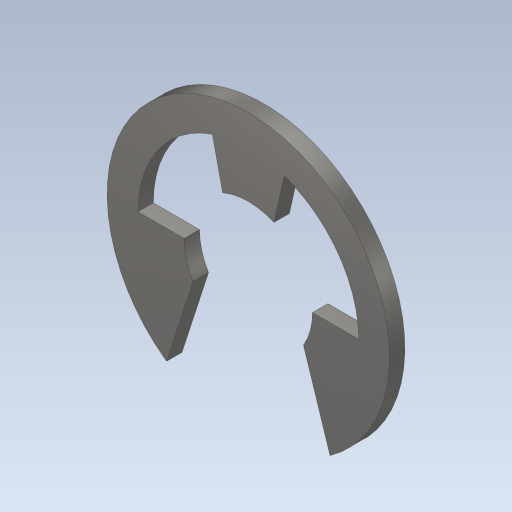
# Autodesk Inventor part: RRING_E_EXT-S-5
Saved by Autodesk Inventor 2024 (Build 280153000, 153)
## iProperties
Created: 2023-10-14
Part Number: RRING_E_EXT-S-5
Material: ステンレス鋼
Catalog Web Link: www.cadenas.de
Description: RRING_E_EXT-Retaining Rings - E
Vendor: MISUMI
Document SubType Name: Modeling
Designer: psAdmin
Manufacturer: MISUMI
Mass: 0.205469 g
Surface Area: 1.19896 cm^2
Volume: 0.0256836 cm^3
Density: 8 g/cm^3
Appearance: 半つや出し
Category: PARTsolutions
Company: MISUMI
PSOL_IDENT_0: {$CADENAS_DATA/23d-libs/misumi/metric/accessories/rring_e_ext.prj},178 {VTYP=3D},{NB=RRING_E_EXT-S-5
PSOL_IDENT_1: },{LINA=RRING_E_EXT-S-5},{NN=RRING_E_EXT},{DATE=08.06.2021 06:39:29},{GEOMDATE=29.08.2013 00:00:00},
PSOL_IDENT_2: {VERSION=},{LINEID=70},{WBVAR=MAT},{WBNUMERIC=}  {NB=RRING_E_EXT-S-5},{LINA=RRING_E_EXT-S-5},{KT=DUM
PSOL_IDENT_3: MY},{PN=RRING_E_EXT-S-5},{TS=RRING_E_EXT},{MAT=-S},{HARD=37~44HRC},{ST=-},{NO=5},{DD=5.0},{DDTOL=0/-
PSOL_IDENT_4: 0.12},{D=11},{DTOL=+0.2/-0.2},{H=4.3},{HTOL=0/-0.30},{TT=0.6},{TTTOL=+0.4/-0.4},{DD1=6~},{LESS=~8},{
PSOL_IDENT_5: DD2=5.0},{DD2TOL=+0.075/0},{MM=0.7},{MMTOL=+0.1/0},{NN=1.2},{MATRR=Steel for Springs},{D1=8.600},{H1=
PSOL_IDENT_6: 2.800},{DEG1=25.400},{DEG2=35.700}
NB: RRING_E_EXT-S-5
NN: 1.2
NT: Retaining Rings - E
NBSYN: $PN.
LINA: RRING_E_EXT-S-5
CATALOG: Misumi
PN: RRING_E_EXT-S-5
MAT: 304 Stainless Steel
HARD: 37~44HRC
ST: -
NO: 5
DD: 5
DDTOL: 0/-0.12
D: 11
DTOL: +0.2/-0.2
H: 4.3
HTOL: 0/-0.30
TT: 0.6
TTTOL: +0.4/-0.4
DD1: 6~
LESS: ~8
DD2: 5
DD2TOL: +0.075/0
MM: 0.7
MMTOL: +0.1/0
SUPPLIER: MISUMI
ARTICLENO: RRING_E_EXT-S-5
BOMINFO: RRING_E_EXT-S-5
CREATOR: CADENAS GmbH
Title: RRING_E_EXT-S-5
Author: Cadenas PARTsolutions
Comments: Retaining Rings - E
Autodesk Inventor part; units mm, degrees
sketch "Sketch_1" plane through (0, 0, 0) normal (0, 0, 1) x (1, 0, 0)
  arc A0 (3.1835, -4.485) -> (-3.1835, -4.485) centre (0, 0) ccw
  line L0 (-3.1835, -4.485) -> (-2.15, -1.2757)
  arc A1 (-2.5, 0) -> (-2.15, -1.2757) centre (0, 0) ccw
  line L1 (-2.5, 0) -> (-4.3, 0)
  arc A2 (-1.4, 4.0657) -> (-4.3, 0) centre (0, 0) ccw
  line L2 (-1.4, 4.0657) -> (-1.0001, 2.2912)
  arc A3 (1.0001, 2.2912) -> (-1.0001, 2.2912) centre (0, 0) ccw
  line L3 (1.0001, 2.2912) -> (1.4, 4.0657)
  arc A4 (4.3, 0) -> (1.4, 4.0657) centre (0, 0) ccw
  line L4 (4.3, 0) -> (2.5, 0)
  arc A5 (2.15, -1.2757) -> (2.5, 0) centre (0, 0) ccw
  line L5 (2.15, -1.2757) -> (3.1835, -4.485)
  constraints: 12 end point, 12 point on circle, 6 centre point
extrude "Extrusion1" add sketch "Sketch_1" along normal mid plane 0.6
ref_plane "COMBINATION_MODULE_XY" through (0, 0, 0.3) normal (0, 0, 1) x (1, 0, 0)
ref_plane "COMBINATION_MODULE_YZ" through (0, 0, 0.3) normal (1, 0, 0) x (0, 1, 0)
ref_plane "COMBINATION_MODULE_ZX" through (0, 0, 0.3) normal (0, 1, 0) x (0, 0, 1)
ref_plane "ring_to_screw_XY" through (0, 0, 0) normal (0, 0, 1) x (1, 0, 0)
ref_plane "ring_to_screw_YZ" through (0, 0, 0) normal (1, 0, 0) x (0, 1, 0)
ref_plane "ring_to_screw_ZX" through (0, 0, 0) normal (0, 1, 0) x (0, 0, 1)
body "Solid1"
